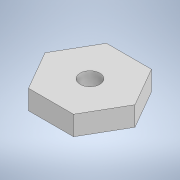
# Autodesk Inventor part: InstruumentarBaraban
Saved by Autodesk Inventor 2022 (Build 260153000, 153)
## iProperties
Created: 2023-08-16
Part Number: InstruumentarBaraban
Material: Generic
Document SubType Name: Modeling
Designer: Kippi
Density: 1 g/cm^3
Appearance: Default
Author: Kippi
Autodesk Inventor part; units mm, degrees
ref_plane "YZ Plane" through (0, 0, 0) normal (1, 0, 0) x (0, 1, 0)
ref_plane "XZ Plane" through (0, 0, 0) normal (0, 1, 0) x (-1, 0, 0)
ref_plane "XY Plane" through (0, 0, 0) normal (0, 0, 1) x (1, 0, 0)
sketch "Sketch1" plane through (0, 0, 0) normal (0, 1, 0) x (-1, 0, 0)
  line L0 (-115.4701, 0) -> (-57.735, 100)
  line L1 (-57.735, 100) -> (57.735, 100)
  line L2 (57.735, 100) -> (115.4701, 0)
  line L3 (115.4701, 0) -> (57.735, -100)
  line L4 (57.735, -100) -> (-57.735, -100)
  line L5 (-57.735, -100) -> (-115.4701, 0)
  circle A0 centre (0, 0) radius 25.2389
  dimension "d0" = 100
  constraints: 12 end point, 2 coincident, 1 centre point, 13 other
  measures "d0" distance from line of L4 point (0, 0)
extrude "Extrusion1" add sketch "Sketch1" along normal blind 50
body "Solid1"
